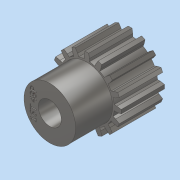
# Autodesk Inventor part: smallIdlerPinion
Saved by Autodesk Inventor 2017 (Build 210142000, 142)
## iProperties
Created: 2016-11-30
Part Number: smallIdlerPinion
Material: Steel, Carbon
Document SubType Name: Modeling
Designer: techn
Density: 7.85 g/cm^3
Appearance: Semi-Polished
Author: techn
Comments: 16 Tooth Traxxas Pinion Gear
Autodesk Inventor part; units mm, degrees
ref_plane "YZ Plane" through (0, 0, 0) normal (1, 0, 0) x (0, 1, 0)
ref_plane "XZ Plane" through (0, 0, 0) normal (0, 1, 0) x (-1, 0, 0)
ref_plane "XY Plane" through (0, 0, 0) normal (0, 0, 1) x (1, 0, 0)
sketch "Sketch1" plane through (0, 0, 0) normal (0, 0, 1) x (1, 0, 0)
  circle A0 centre (0, 0) radius 4.7371
  dimension "d0" = 9.4742
  constraints: 1 centre point, 1 coincident
  measures "d0" diameter of A0
extrude "Extrusion1" add sketch "Sketch1" along normal blind 5.969
sketch "Sketch2" plane through (0, 0, 5.969) normal (0, 0, 1) x (1, 0, 0)
  circle A0 centre (0, 0) radius 3.556
  dimension "d3" = 7.112
  constraints: 1 centre point, 1 coincident
  measures "d3" diameter of A0
extrude "Extrusion2" add sketch "Sketch2" along normal blind 5.08
sketch "Sketch3" plane through (0, 0, 11.049) normal (0, 0, 1) x (1, 0, 0)
  circle A0 centre (0, 0) radius 1.5875
  dimension "d6" = 3.175
  constraints: 1 centre point, 1 coincident
  measures "d6" diameter of A0
extrude "Extrusion3" cut sketch "Sketch3" against normal blind 25.4
sketch "Sketch4" plane through (0, 0, 0) normal (0, 0, -1) x (-1, 0, 0)
  circle A0 centre (0, 0) radius 3.7821
  line L0 (0.3624, 3.7647) -> (0.3624, 4.1457)
  line L1 (-0.3624, 3.7647) -> (-0.3624, 4.1457)
  line L2 (-0.3624, 4.1457) -> (-0.2617, 4.7299)
  line L3 (-0.2617, 4.7299) -> (0.2617, 4.7299)
  line L4 (0.2617, 4.7299) -> (0.3624, 4.1457)
  line L5 (-0.3624, 3.7647) -> (0.3624, 3.7647)
  line L6 (-1.7755, 3.3394) -> (-1.9213, 3.6914)
  line L7 (-1.9213, 3.6914) -> (-2.0518, 4.2697)
  line L8 (-2.0518, 4.2697) -> (-1.5682, 4.47)
  line L9 (-1.5682, 4.47) -> (-1.2517, 3.9688)
  line L10 (-1.1059, 3.6168) -> (-1.2517, 3.9688)
  line L11 (-1.7755, 3.3394) -> (-1.1059, 3.6168)
  line L12 (-2.9183, 2.4058) -> (-3.1877, 2.6752)
  line L13 (-3.1877, 2.6752) -> (-3.5296, 3.1595)
  line L14 (-3.5296, 3.1595) -> (-3.1595, 3.5296)
  line L15 (-3.1595, 3.5296) -> (-2.6752, 3.1877)
  line L16 (-2.4058, 2.9183) -> (-2.6752, 3.1877)
  line L17 (-2.9183, 2.4058) -> (-2.4058, 2.9183)
  line L18 (-3.6168, 1.1059) -> (-3.9688, 1.2517)
  line L19 (-3.9688, 1.2517) -> (-4.47, 1.5682)
  line L20 (-4.47, 1.5682) -> (-4.2697, 2.0518)
  line L21 (-4.2697, 2.0518) -> (-3.6914, 1.9213)
  line L22 (-3.3394, 1.7755) -> (-3.6914, 1.9213)
  line L23 (-3.6168, 1.1059) -> (-3.3394, 1.7755)
  line L24 (-3.7647, -0.3624) -> (-4.1457, -0.3624)
  line L25 (-4.1457, -0.3624) -> (-4.7299, -0.2617)
  line L26 (-4.7299, -0.2617) -> (-4.7299, 0.2617)
  line L27 (-4.7299, 0.2617) -> (-4.1457, 0.3624)
  line L28 (-3.7647, 0.3624) -> (-4.1457, 0.3624)
  line L29 (-3.7647, -0.3624) -> (-3.7647, 0.3624)
  line L30 (-3.3394, -1.7755) -> (-3.6914, -1.9213)
  line L31 (-3.6914, -1.9213) -> (-4.2697, -2.0518)
  line L32 (-4.2697, -2.0518) -> (-4.47, -1.5682)
  line L33 (-4.47, -1.5682) -> (-3.9688, -1.2517)
  line L34 (-3.6168, -1.1059) -> (-3.9688, -1.2517)
  line L35 (-3.3394, -1.7755) -> (-3.6168, -1.1059)
  line L36 (-2.4058, -2.9183) -> (-2.6752, -3.1877)
  line L37 (-2.6752, -3.1877) -> (-3.1595, -3.5296)
  line L38 (-3.1595, -3.5296) -> (-3.5296, -3.1595)
  line L39 (-3.5296, -3.1595) -> (-3.1877, -2.6752)
  line L40 (-2.9183, -2.4058) -> (-3.1877, -2.6752)
  line L41 (-2.4058, -2.9183) -> (-2.9183, -2.4058)
  line L42 (-1.1059, -3.6168) -> (-1.2517, -3.9688)
  line L43 (-1.2517, -3.9688) -> (-1.5682, -4.47)
  line L44 (-1.5682, -4.47) -> (-2.0518, -4.2697)
  line L45 (-2.0518, -4.2697) -> (-1.9213, -3.6914)
  line L46 (-1.7755, -3.3394) -> (-1.9213, -3.6914)
  line L47 (-1.1059, -3.6168) -> (-1.7755, -3.3394)
  line L48 (0.3624, -3.7647) -> (0.3624, -4.1457)
  line L49 (0.3624, -4.1457) -> (0.2617, -4.7299)
  line L50 (0.2617, -4.7299) -> (-0.2617, -4.7299)
  line L51 (-0.2617, -4.7299) -> (-0.3624, -4.1457)
  line L52 (-0.3624, -3.7647) -> (-0.3624, -4.1457)
  line L53 (0.3624, -3.7647) -> (-0.3624, -3.7647)
  line L54 (1.7755, -3.3394) -> (1.9213, -3.6914)
  line L55 (1.9213, -3.6914) -> (2.0518, -4.2697)
  line L56 (2.0518, -4.2697) -> (1.5682, -4.47)
  line L57 (1.5682, -4.47) -> (1.2517, -3.9688)
  line L58 (1.1059, -3.6168) -> (1.2517, -3.9688)
  line L59 (1.7755, -3.3394) -> (1.1059, -3.6168)
  line L60 (2.9183, -2.4058) -> (3.1877, -2.6752)
  line L61 (3.1877, -2.6752) -> (3.5296, -3.1595)
  line L62 (3.5296, -3.1595) -> (3.1595, -3.5296)
  line L63 (3.1595, -3.5296) -> (2.6752, -3.1877)
  line L64 (2.4058, -2.9183) -> (2.6752, -3.1877)
  line L65 (2.9183, -2.4058) -> (2.4058, -2.9183)
  line L66 (3.6168, -1.1059) -> (3.9688, -1.2517)
  line L67 (3.9688, -1.2517) -> (4.47, -1.5682)
  line L68 (4.47, -1.5682) -> (4.2697, -2.0518)
  line L69 (4.2697, -2.0518) -> (3.6914, -1.9213)
  line L70 (3.3394, -1.7755) -> (3.6914, -1.9213)
  line L71 (3.6168, -1.1059) -> (3.3394, -1.7755)
  line L72 (3.7647, 0.3624) -> (4.1457, 0.3624)
  line L73 (4.1457, 0.3624) -> (4.7299, 0.2617)
  line L74 (4.7299, 0.2617) -> (4.7299, -0.2617)
  line L75 (4.7299, -0.2617) -> (4.1457, -0.3624)
  line L76 (3.7647, -0.3624) -> (4.1457, -0.3624)
  line L77 (3.7647, 0.3624) -> (3.7647, -0.3624)
  line L78 (3.3394, 1.7755) -> (3.6914, 1.9213)
  line L79 (3.6914, 1.9213) -> (4.2697, 2.0518)
  line L80 (4.2697, 2.0518) -> (4.47, 1.5682)
  line L81 (4.47, 1.5682) -> (3.9688, 1.2517)
  line L82 (3.6168, 1.1059) -> (3.9688, 1.2517)
  line L83 (3.3394, 1.7755) -> (3.6168, 1.1059)
  line L84 (2.4058, 2.9183) -> (2.6752, 3.1877)
  line L85 (2.6752, 3.1877) -> (3.1595, 3.5296)
  line L86 (3.1595, 3.5296) -> (3.5296, 3.1595)
  line L87 (3.5296, 3.1595) -> (3.1877, 2.6752)
  line L88 (2.9183, 2.4058) -> (3.1877, 2.6752)
  line L89 (2.4058, 2.9183) -> (2.9183, 2.4058)
  line L90 (1.1059, 3.6168) -> (1.2517, 3.9688)
  line L91 (1.2517, 3.9688) -> (1.5682, 4.47)
  line L92 (1.5682, 4.47) -> (2.0518, 4.2697)
  line L93 (2.0518, 4.2697) -> (1.9213, 3.6914)
  line L94 (1.7755, 3.3394) -> (1.9213, 3.6914)
  line L95 (1.1059, 3.6168) -> (1.7755, 3.3394)
  circle A1 centre (0, 0) radius 4.7556
  circle A2 centre (0, 0) radius 4.7371 projected
  dimension "d10" = 0.381
  dimension "d13" = 360
  dimension "d20" = 0.5234
  dimension "d21" = 0.7247
  dimension "d23" = 0.9652
  constraints: 192 end point, 2 centre point, 2 coincident, 2 equal length, 2 point on circle, 2 vertical, 1 horizontal, 1 perpendicular, 195 other
  measures "d10" distance of L0.start L0.end
  measures "d20" distance of L2.end L3.end
  measures "d21" distance of L1.start L0.start
  measures "d23" distance from line of L1.start L3
extrude "Extrusion4" cut sketch "Sketch4" against normal up to surface (5.969 mm away) contours A0 L82 L81 A2 L73 L72 | L76 L75 A2 L67 L66 A0 | A0 L88 L87 A2 L79 L78 | A2 L74 | L70 L69 A2 L61 L60 A0 | L80 A2 | A2 L68 | A0 L94 L93 A2 L85 L84 | L64 L63 A2 L55 L54 A0 | L86 A2 | A2 L62 | A0 L0 L4 A2 L91 L90 | L58 L57 A2 L49 L48 A0 | L92 A2 | A2 L56 | A0 L10 L9 A2 L2 L1 | L52 L51 A2 L43 L42 A0 | L3 A2 | A2 L50 | A0 L16 L15 A2 L7 L6 | L46 L45 A2 L37 L36 A0 | L8 A2 | A2 L44 | A0 L22 L21 A2 L13 L12 | L40 L39 A2 L31 L30 A0 | L14 A2 | A2 L38 | A0 L28 L27 A2 L19 L18 | L34 L33 A2 L25 L24 A0 | L20 A2 | A2 L32 | L26 A2 | A1
sketch "Sketch6" plane through (0, 0, 11.049) normal (0, 0, 1) x (1, 0, 0)
  line L0 (-2.7388, -2.1365) -> (-2.7388, 2.0332) construction
  line L1 (-2.7388, 2.0332) -> (-1.8007, 2.0332) construction
  line L2 (-1.8007, 2.0332) -> (-1.8007, -2.1365) construction
  line L3 (-1.8007, -2.1365) -> (-2.7388, -2.1365) construction
  line L4 (-1.8847, -1.6025) -> (-1.8847, -2.0099)
  line L5 (-1.8847, -2.0099) -> (-1.9699, -2.0099)
  line L6 (-1.9699, -2.0099) -> (-1.9699, -1.8583)
  line L7 (-1.9699, -1.8583) -> (-2.5296, -1.8583)
  line L8 (-2.5296, -1.8583) -> (-2.5296, -2.0099)
  line L9 (-2.5296, -2.0099) -> (-2.6061, -2.0099)
  spline S0 degree 2 poles (-2.6061, -2.0099) (-2.6061, -1.924) (-2.6548, -1.8428) (-2.7225, -1.8373) knots 0 0 0 1 2 2 2
  line L10 (-2.7225, -1.8373) -> (-2.7225, -1.7507)
  line L11 (-2.7225, -1.7507) -> (-1.9699, -1.7507)
  line L12 (-1.9699, -1.7507) -> (-1.9699, -1.6025)
  line L13 (-1.9699, -1.6025) -> (-1.8847, -1.6025)
  spline S1 degree 2 poles (-2.1554, -0.921) (-2.0911, -0.921) (-1.9821, -0.9636) (-1.9456, -0.9995) knots 0 0 0 1 2 2 2
  spline S2 degree 2 poles (-1.9456, -0.9995) (-1.907, -1.0367) (-1.8671, -1.1301) (-1.8671, -1.1863) knots 0 0 0 1 2 2 2
  spline S3 degree 2 poles (-1.8671, -1.1863) (-1.8671, -1.2424) (-1.905, -1.3352) (-1.9429, -1.3704) knots 0 0 0 1 2 2 2
  spline S4 degree 2 poles (-1.9429, -1.3704) (-1.9882, -1.4137) (-2.1405, -1.4624) (-2.2515, -1.4624) knots 0 0 0 1 2 2 2
  spline S5 degree 2 poles (-2.2515, -1.4624) (-2.3604, -1.4624) (-2.5357, -1.4177) (-2.6007, -1.371) knots 0 0 0 1 2 2 2
  spline S6 degree 2 poles (-2.6007, -1.371) (-2.6643, -1.3257) (-2.7354, -1.1822) (-2.7354, -1.0881) knots 0 0 0 1 2 2 2
  spline S7 degree 2 poles (-2.7354, -1.0881) (-2.7354, -1.0604) (-2.73, -1.0117) (-2.7239, -0.9934) knots 0 0 0 1 2 2 2
  line L14 (-2.7239, -0.9934) -> (-2.6163, -0.9934)
  line L15 (-2.6163, -0.9934) -> (-2.6163, -0.9981)
  spline S8 degree 2 poles (-2.6163, -0.9981) (-2.6244, -1.0137) (-2.6386, -1.0705) (-2.6386, -1.103) knots 0 0 0 1 2 2 2
  spline S9 degree 2 poles (-2.6386, -1.103) (-2.6386, -1.2073) (-2.4978, -1.3352) (-2.3598, -1.3473) knots 0 0 0 1 2 2 2
  spline S10 degree 2 poles (-2.3598, -1.3473) (-2.3875, -1.3074) (-2.418, -1.2235) (-2.418, -1.1734) knots 0 0 0 1 2 2 2
  spline S11 degree 2 poles (-2.418, -1.1734) (-2.418, -1.1247) (-2.3983, -1.0516) (-2.3686, -1.0117) knots 0 0 0 1 2 2 2
  spline S12 degree 2 poles (-2.3686, -1.0117) (-2.334, -0.9656) (-2.2271, -0.921) (-2.1554, -0.921) knots 0 0 0 1 2 2 2
  spline S13 degree 2 poles (-2.1506, -1.0347) (-2.2021, -1.0347) (-2.2718, -1.0617) (-2.2961, -1.0915) knots 0 0 0 1 2 2 2
  spline S14 degree 2 poles (-2.2961, -1.0915) (-2.3137, -1.1139) (-2.3252, -1.1694) (-2.3252, -1.1985) knots 0 0 0 1 2 2 2
  spline S15 degree 2 poles (-2.3252, -1.1985) (-2.3252, -1.2377) (-2.3016, -1.3115) (-2.2792, -1.3473) knots 0 0 0 1 2 2 2
  spline S16 degree 2 poles (-2.2792, -1.3473) (-2.267, -1.348) (-2.244, -1.3494) (-2.2264, -1.3494) knots 0 0 0 1 2 2 2
  spline S17 degree 2 poles (-2.2264, -1.3494) (-2.1398, -1.3494) (-2.0336, -1.3155) (-2.0058, -1.2898) knots 0 0 0 1 2 2 2
  spline S18 degree 2 poles (-2.0058, -1.2898) (-1.9794, -1.2661) (-1.9584, -1.2147) (-1.9584, -1.1856) knots 0 0 0 1 2 2 2
  spline S19 degree 2 poles (-1.9584, -1.1856) (-1.9584, -1.1179) (-2.0545, -1.0347) (-2.1506, -1.0347) knots 0 0 0 1 2 2 2
  line L16 (-1.8847, -0.6036) -> (-2.621, -0.6036)
  line L17 (-2.621, -0.6036) -> (-2.621, -0.8838)
  line L18 (-2.621, -0.8838) -> (-2.7198, -0.8838)
  line L19 (-2.7198, -0.8838) -> (-2.7198, -0.2124)
  line L20 (-2.7198, -0.2124) -> (-2.621, -0.2124)
  line L21 (-2.621, -0.2124) -> (-2.621, -0.4926)
  line L22 (-2.621, -0.4926) -> (-1.8847, -0.4926)
  line L23 (-1.8847, -0.4926) -> (-1.8847, -0.6036)
  line L24 (-2.1716, 0.7446) -> (-2.1716, 0.6451)
  line L25 (-2.1716, 0.6451) -> (-1.8847, 0.6451)
  line L26 (-1.8847, 0.6451) -> (-1.8847, 0.5375)
  line L27 (-1.8847, 0.5375) -> (-2.1716, 0.5375)
  line L28 (-2.1716, 0.5375) -> (-2.1716, 0.1686)
  line L29 (-2.1716, 0.1686) -> (-2.2894, 0.1686)
  line L30 (-2.2894, 0.1686) -> (-2.7198, 0.5422)
  line L31 (-2.7198, 0.5422) -> (-2.7198, 0.6451)
  line L32 (-2.7198, 0.6451) -> (-2.2616, 0.6451)
  line L33 (-2.2616, 0.6451) -> (-2.2616, 0.7446)
  line L34 (-2.2616, 0.7446) -> (-2.1716, 0.7446)
  line L35 (-2.2616, 0.5375) -> (-2.5878, 0.5375)
  line L36 (-2.5878, 0.5375) -> (-2.2616, 0.2566)
  line L37 (-2.2616, 0.2566) -> (-2.2616, 0.5375)
  spline S20 degree 2 poles (-1.8657, 1.0864) (-1.8657, 1.0241) (-1.9029, 0.9219) (-1.9374, 0.886) knots 0 0 0 1 2 2 2
  spline S21 degree 2 poles (-1.9374, 0.886) (-1.9713, 0.8508) (-2.0633, 0.8143) (-2.1154, 0.8143) knots 0 0 0 1 2 2 2
  spline S22 degree 2 poles (-2.1154, 0.8143) (-2.1831, 0.8143) (-2.2968, 0.8867) (-2.3307, 0.9557) knots 0 0 0 1 2 2 2
  line L38 (-2.3307, 0.9557) -> (-2.334, 0.9557)
  spline S23 degree 2 poles (-2.334, 0.9557) (-2.3699, 0.8942) (-2.4552, 0.8346) (-2.5188, 0.8346) knots 0 0 0 1 2 2 2
  spline S24 degree 2 poles (-2.5188, 0.8346) (-2.6129, 0.8346) (-2.7388, 0.9767) (-2.7388, 1.0864) knots 0 0 0 1 2 2 2
  spline S25 degree 2 poles (-2.7388, 1.0864) (-2.7388, 1.2001) (-2.6196, 1.3375) (-2.5263, 1.3375) knots 0 0 0 1 2 2 2
  spline S26 degree 2 poles (-2.5263, 1.3375) (-2.4701, 1.3375) (-2.3604, 1.2718) (-2.3293, 1.2102) knots 0 0 0 1 2 2 2
  line L39 (-2.3293, 1.2102) -> (-2.3259, 1.2102)
  spline S27 degree 2 poles (-2.3259, 1.2102) (-2.2921, 1.2833) (-2.1946, 1.3584) (-2.1175, 1.3584) knots 0 0 0 1 2 2 2
  spline S28 degree 2 poles (-2.1175, 1.3584) (-2.0105, 1.3584) (-1.8657, 1.2028) (-1.8657, 1.0864) knots 0 0 0 1 2 2 2
  spline S29 degree 2 poles (-2.1066, 1.2434) (-2.1581, 1.2434) (-2.219, 1.2028) (-2.2501, 1.1452) knots 0 0 0 1 2 2 2
  spline S30 degree 2 poles (-2.2501, 1.1452) (-2.261, 1.1263) (-2.286, 1.0627) (-2.3022, 1.0228) knots 0 0 0 1 2 2 2
  spline S31 degree 2 poles (-2.3022, 1.0228) (-2.2718, 0.9767) (-2.1811, 0.9273) (-2.1236, 0.9273) knots 0 0 0 1 2 2 2
  spline S32 degree 2 poles (-2.1236, 0.9273) (-2.0478, 0.9273) (-1.949, 1.0187) (-1.949, 1.0877) knots 0 0 0 1 2 2 2
  spline S33 degree 2 poles (-1.949, 1.0877) (-1.949, 1.1581) (-2.0336, 1.2434) (-2.1066, 1.2434) knots 0 0 0 1 2 2 2
  spline S34 degree 2 poles (-2.5249, 1.2278) (-2.5811, 1.2278) (-2.6562, 1.1527) (-2.6562, 1.0857) knots 0 0 0 1 2 2 2
  spline S35 degree 2 poles (-2.6562, 1.0857) (-2.6562, 1.0248) (-2.5892, 0.947) (-2.5317, 0.947) knots 0 0 0 1 2 2 2
  spline S36 degree 2 poles (-2.5317, 0.947) (-2.4904, 0.947) (-2.4329, 0.9869) (-2.4098, 1.0268) knots 0 0 0 1 2 2 2
  spline S37 degree 2 poles (-2.4098, 1.0268) (-2.4004, 1.0437) (-2.3672, 1.1155) (-2.3577, 1.1446) knots 0 0 0 1 2 2 2
  spline S38 degree 2 poles (-2.3577, 1.1446) (-2.395, 1.1933) (-2.4741, 1.2278) (-2.5249, 1.2278) knots 0 0 0 1 2 2 2
  spline S39 degree 2 poles (-2.468, 2.0122) (-2.4139, 2.0122) (-2.3164, 1.9736) (-2.2826, 1.9391) knots 0 0 0 1 2 2 2
  spline S40 degree 2 poles (-2.2826, 1.9391) (-2.24, 1.8958) (-2.196, 1.7787) (-2.196, 1.6894) knots 0 0 0 1 2 2 2
  line L40 (-2.196, 1.6894) -> (-2.196, 1.5953)
  line L41 (-2.196, 1.5953) -> (-1.8847, 1.5953)
  line L42 (-1.8847, 1.5953) -> (-1.8847, 1.4843)
  line L43 (-1.8847, 1.4843) -> (-2.7198, 1.4843)
  line L44 (-2.7198, 1.4843) -> (-2.7198, 1.6941)
  spline S41 degree 2 poles (-2.7198, 1.6941) (-2.7198, 1.7686) (-2.6954, 1.8728) (-2.6677, 1.9127) knots 0 0 0 1 2 2 2
  spline S42 degree 2 poles (-2.6677, 1.9127) (-2.6359, 1.9594) (-2.5378, 2.0122) (-2.468, 2.0122) knots 0 0 0 1 2 2 2
  spline S43 degree 2 poles (-2.4647, 1.8965) (-2.508, 1.8965) (-2.5716, 1.8667) (-2.5919, 1.8362) knots 0 0 0 1 2 2 2
  spline S44 degree 2 poles (-2.5919, 1.8362) (-2.6095, 1.8099) (-2.6237, 1.7395) (-2.6237, 1.6874) knots 0 0 0 1 2 2 2
  line L45 (-2.6237, 1.6874) -> (-2.6237, 1.5953)
  line L46 (-2.6237, 1.5953) -> (-2.2907, 1.5953)
  line L47 (-2.2907, 1.5953) -> (-2.2907, 1.6711)
  spline S45 degree 2 poles (-2.2907, 1.6711) (-2.2907, 1.7388) (-2.3124, 1.822) (-2.3408, 1.8491) knots 0 0 0 1 2 2 2
  spline S46 degree 2 poles (-2.3408, 1.8491) (-2.3659, 1.8741) (-2.4247, 1.8965) (-2.4647, 1.8965) knots 0 0 0 1 2 2 2
  point P0 (0, 0)
  dimension "d3" = 7.112
  constraints: 2 other
emboss "Emboss2" sketch "Sketch6" operation cut depth 0.254 direction (0, 0, -1)
body "Solid1"
